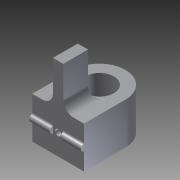
# Autodesk Inventor part: LaserMountTop
Saved by Autodesk Inventor 2011 (Build 150239000, 239)
## iProperties
Created: 2010-07-18
Part Number: LaserMountTop
Document SubType Name: Modeling
Designer: abarry
Density: 1 g/cm^3
Author: abarry
Autodesk Inventor part; units mm, degrees
ref_plane "YZ Plane" through (0, 0, 0) normal (1, 0, 0) x (0, 1, 0)
ref_plane "XZ Plane" through (0, 0, 0) normal (0, 1, 0) x (-1, 0, 0)
ref_plane "XY Plane" through (0, 0, 0) normal (0, 0, 1) x (1, 0, 0)
sketch "Sketch1" plane through (0, 0, 0) normal (0, 0, 1) x (1, 0, 0)
  circle A0 centre (0, 0) radius 7
  arc A1 (12.5, 0) -> (-12.5, 0) centre (0, 0) ccw
  line L0 (-12.5, 0) -> (-12.5, -20)
  line L1 (12.5, 0) -> (12.5, -20)
  line L2 (12.5, -20) -> (-12.5, -20)
  dimension "d0" = 14
  dimension "d1" = 25
  dimension "d2" = 20
  constraints: 6 end point, 2 centre point, 2 coincident, 2 point on circle, 2 tangent, 1 parallel, 1 perpendicular, 1 vertical
  measures "d0" diameter of A0
  measures "d1" diameter of A1
  measures "d2" distance of L0.start L0.end
extrude "Main Extrusion" add sketch "Sketch1" along normal blind 20
sketch "Sketch2" plane through (-12.5, -20, 0) normal (0, -1, 0) x (1, 0, 0)
  line L0 (25, 20) -> (0, 20) projected
  line L1 (0, 0) -> (0, 20) projected
  line L2 (25, 0) -> (0, 0) projected
  line L3 (25, 0) -> (25, 20) projected
  line L4 (0, 10) -> (25, 10) construction
  line L5 (12.5, 20) -> (12.5, 0) construction
  circle A0 centre (12.5, 10) radius 1.5
  dimension "d5" = 3
  constraints: 4 end point, 4 midpoint, 1 centre point, 1 perpendicular
  measures "d5" diameter of A0
extrude "Mount Pivot Hole" cut sketch "Sketch2" against normal blind 10 contours A0
sketch "Sketch3" plane through (0, 0, 20) normal (0, 0, 1) x (1, 0, 0)
  line L0 (12.5, -20) -> (-12.5, -20) construction
  line L1 (-2.5, -20) -> (-2.5, -8)
  line L2 (-2.5, -8) -> (2.5, -8)
  line L3 (2.5, -8) -> (2.5, -20)
  line L4 (-12.5, -20) -> (-12.5, 0) construction
  line L5 (12.5, 0) -> (12.5, -20) construction
  line L6 (-2.5, -15.4171) -> (-12.5, -15.4171) construction
  line L7 (2.5, -15.4171) -> (12.5, -15.4171) construction
  line L8 (-2.5, -20) -> (2.5, -20)
  dimension "d8" = 12
  dimension "d9" = 5
  constraints: 12 end point, 6 point on line, 5 perpendicular, 2 collinear
  measures "d8" distance of L1.start L1.end
  measures "d9" distance of L1.end L2.end
extrude "Handle" add sketch "Sketch3" along normal blind 20
fillet "Fillet1" radius 5 2 edges at (-2.5, -14, 20) (2.5, -14, 20)
fillet "Fillet2" radius 2 3 edges at (-5, -8, 20) (0, -8, 20) (5, -8, 20)
sketch "Sketch8" plane through (-12.5, -20, 0) normal (-1, 0, 0) x (0, 0, 1)
  line L0 (0, 0) -> (20, 0) projected
  arc A0 (8.5, 0) -> (11.5, 0) centre (10, 0) ccw
  point P0 (0, 20)
  dimension "d21" = 1.5
  constraints: 2 point on circle, 2 point on line, 1 centre point, 1 coincident, 1 midpoint
  measures "d21" radius of A0
extrude "Notch Right" add sketch "Sketch8" against normal blind 10
sketch "Sketch9" plane through (12.5, -20, 0) normal (1, 0, 0) x (0, 0, -1)
  arc A0 (-11.5, 0) -> (-8.5, 0) centre (-10, 0) ccw projected
  line L0 (-11.5, 0) -> (-8.5, 0) projected
  point P0 (0, 20)
extrude "Notch Left" add sketch "Sketch9" against normal blind 10
fillet "Fillet3" radius 1 4 edges at (-7.5, -20, 11.5) (-7.5, -20, 8.5) (7.5, -20, 11.5) (7.5, -20, 8.5)
sketch "Sketch5" plane through (-12.5, -20, 0) normal (-1, 0, 0) x (0, 0, 1)
  line L0 (0, 0) -> (20, 0) projected
  arc A0 (11, 0) -> (9, 0) centre (10, 0) ccw
  point P0 (0, 20)
  dimension "d16" = 1
  constraints: 2 point on circle, 2 point on line, 1 centre point, 1 coincident, 1 midpoint
  measures "d16" radius of A0
sketch "Sketch6" plane through (12.5, -20, 0) normal (1, 0, 0) x (0, 0, -1)
  line L0 (0, 0) -> (-20, 0) projected
  arc A0 (-9, 0) -> (-11, 0) centre (-10, 0) ccw projected
  point P0 (0, 20)
  dimension "d14" = 1
  dimension "d15" = 7.5
  constraints: 20 end point, 5 point on line, 4 parallel, 3 equal length, 3 perpendicular, 2 horizontal, 1 collinear, 1 midpoint, 1 vertical
body "Solid1"
